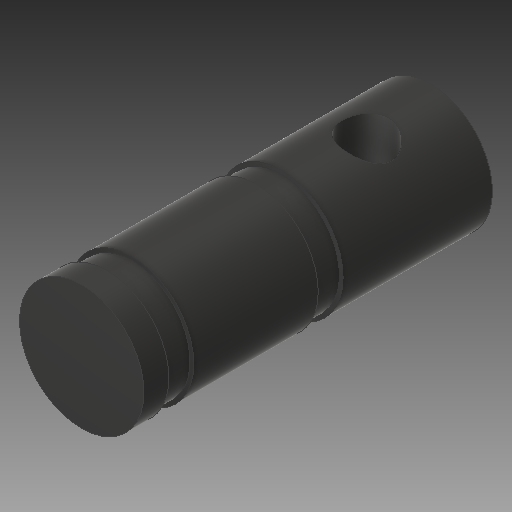
# Autodesk Inventor part: waleczek_do_sprezyn_fi6
Saved by Autodesk Inventor 2017 (Build 210142000, 142)
## iProperties
Created: 2021-05-20
Part Number: waleczek_do_sprezyn_fi6
Material: Generic
Document SubType Name: Modeling
Designer: majch
Density: 1 g/cm^3
Appearance: Smooth - Black
Mass: 0.255209 g
Surface Area: 2.89377 cm^2
Volume: 0.255209 cm^3
Author: majch
Autodesk Inventor part; units mm, degrees
ref_plane "YZ Plane" through (0, 0, 0) normal (1, 0, 0) x (0, 1, 0)
ref_plane "XZ Plane" through (0, 0, 0) normal (0, 1, 0) x (-1, 0, 0)
ref_plane "XY Plane" through (0, 0, 0) normal (0, 0, 1) x (1, 0, 0)
sketch "Sketch2" plane through (0, 0, 0) normal (0, 1, 0) x (-1, 0, 0)
  line L0 (0, 14) -> (2.5, 14)
  line L1 (2.5, 14) -> (2.5, 13)
  line L2 (2.5, 13) -> (2.35, 13)
  line L3 (2.35, 13) -> (2.35, 12)
  line L4 (2.35, 12) -> (2.5, 12)
  line L5 (2.5, 12) -> (2.5, 7)
  line L6 (2.5, 7) -> (2.35, 7)
  line L7 (2.35, 7) -> (2.35, 6)
  line L8 (2.35, 6) -> (2.5, 6)
  line L9 (2.5, 6) -> (2.5, 0)
  line L10 (2.5, 0) -> (0, 0)
  line L11 (0, 14) -> (0, 0)
  dimension "d3" = 2.5
  dimension "d6" = 1
  dimension "d7" = 0.15
  dimension "d8" = 1
  dimension "d9" = 0.15
  dimension "d10" = 5
  dimension "d11" = 0.15
  dimension "d12" = 1
  dimension "d13" = 0.15
  dimension "d15" = 2.5
  dimension "d21" = 14
  constraints: 24 end point, 6 perpendicular, 6 point on line, 1 coincident, 1 vertical
  measures "d3" distance of L0.start L0.end
  measures "d6" distance of L0.end L1.end
  measures "d7" distance of L1.end L2.end
  measures "d8" distance of L2.end L3.end
  measures "d9" distance of L3.end L4.end
  measures "d10" distance of L4.end L5.end
  measures "d11" distance of L5.end L6.end
  measures "d12" distance of L6.end L7.end
  measures "d13" distance of L7.end L8.end
  measures "d15" distance of L9.end L10.end
  measures "d21" distance of L0.start L10.end
revolve "Revolution1" add sketch "Sketch2" angle 360 about axis through (0, 0, 14) along (0, 0, -1)
sketch "Sketch3" plane through (0, 0, 0) normal (0, 1, 0) x (-1, 0, 0)
  circle A0 centre (-0.45, 3) radius 1
  line L0 (-2.5, 0) -> (2.5, 0) projected
  point P0 (0, 0)
  dimension "d17" = 2
  dimension "d18" = 3
  constraints: 1 centre point
  measures "d17" diameter of A0
  measures "d18" distance from line of L0 A0.centre
extrude "Extrusion2" cut sketch "Sketch3" along normal through all both and the other way through all
body "Solid2"
